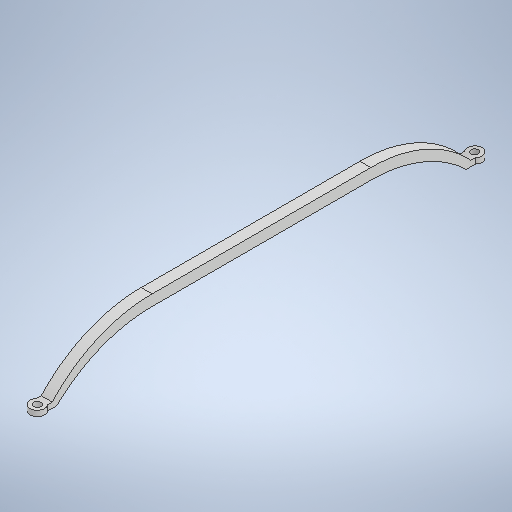
# Autodesk Inventor part: lacznik2
Saved by Autodesk Inventor 2025.2 (Build 292293000, 293)
## iProperties
Created: 2025-05-29
Part Number: lacznik2
Material: Ogólny
Document SubType Name: Modeling
Designer: janla
Density: 1 g/cm^3
Appearance: Domyślna
Author: janla
Autodesk Inventor part; units mm, degrees
ref_plane "YZ Plane" through (0, 0, 0) normal (1, 0, 0) x (0, 1, 0)
ref_plane "XZ Plane" through (0, 0, 0) normal (0, 1, 0) x (-1, 0, 0)
ref_plane "XY Plane" through (0, 0, 0) normal (0, 0, 1) x (1, 0, 0)
sketch "Szkic1" plane through (0, 0, 0) normal (0, 1, 0) x (-1, 0, 0)
  line L0 (0, 0) -> (0, -120)
  line L1 (0, -120) -> (0, 120)
  circle A0 centre (0, 120) radius 2
  circle A1 centre (0, -120) radius 2
  circle A2 centre (0, -120) radius 4
  circle A3 centre (0, 120) radius 4
  line L2 (-3, 117.3542) -> (3, 117.3542)
  line L3 (3, 117.3542) -> (3, -117.3542)
  line L4 (3, -117.3542) -> (-3, -117.3542)
  line L5 (-3, -117.3542) -> (-3, 117.3542)
  line L6 (3, 117.3542) -> (-3, 117.3542)
  line L7 (-3, 117.3542) -> (-3, 112.3542)
  line L8 (-3, 112.3542) -> (3, 112.3542)
  line L9 (3, 112.3542) -> (3, 117.3542)
  line L10 (3, -117.3542) -> (-3, -117.3542)
  line L11 (-3, -117.3542) -> (-3, -112.3542)
  line L12 (-3, -112.3542) -> (3, -112.3542)
  line L13 (3, -112.3542) -> (3, -117.3542)
  point P0 (-3, -117.3542)
  point P1 (3, -112.3542)
  point P2 (3, 112.3542)
  dimension "d4" = 8
  dimension "d5" = 8
  dimension "d0" = 120
  dimension "d1" = 240
  dimension "d2" = 4
  dimension "d3" = 4
  dimension "d6" = 3
  dimension "d7" = 3
  dimension "d14" = 5
  dimension "d15" = 5
  constraints: 28 end point, 6 parallel, 4 coincident, 3 horizontal, 3 perpendicular, 3 point on line, 2 centre point, 1 vertical, 6 other
  measures "d0" distance of L0.start L0.end
  measures "d1" distance of L0.end L1.end
  measures "d2" diameter of A0
  measures "d3" diameter of A1
  measures "d6" distance between parallel lines of L0 L5
  measures "d7" distance between parallel lines of L3 L0
  measures "d14" distance between parallel lines of L8 L2
  measures "d15" distance between parallel lines of L4 L12
extrude "Wyciągnięcie proste1" add sketch "Szkic1" along normal blind 3 contours L12 L3 A2 L0 | L0 A2 L5 L12 | L8 L5 A3 L1 | L1 A3 L3 L8 | A2 L4 L0 | L0 L4 A2 | A3 L2 L1 | L1 L2 A3 | L4 A2 | L2 A3
sketch "Szkic4" plane through (3, 0, 117.3542) normal (1, 0, 0) x (0, 0, -1)
  line L0 (0, 3) -> (5, 3) projected
  line L1 (2.5, 3) -> (232.2085, 3)
  line L2 (232.2085, 3) -> (117.3542, 3)
  line L3 (117.3542, 0) -> (117.3542, 27)
  line L4 (117.3542, 27) -> (177.3542, 27)
  line L5 (177.3542, 27) -> (57.3542, 27)
  arc A0 (57.3542, 27) -> (2.5, 3) centre (57.3542, -47.6873) ccw
  arc A1 (232.2085, 3) -> (177.3542, 27) centre (177.3542, -47.6873) ccw
  line L6 (57.3542, 27) -> (177.3542, 27)
  line L7 (177.3542, 27) -> (177.3542, 21)
  line L8 (177.3542, 21) -> (57.3542, 21)
  line L9 (57.3542, 21) -> (57.3542, 27)
  line L10 (0, 0) -> (5, 0) projected
  arc A2 (57.3542, 21) -> (5, 0) centre (57.3542, -54.7611) ccw
  line L11 (229.7085, 0) -> (229.7085, 3) projected
  arc A3 (229.7085, 0) -> (177.3542, 21) centre (177.3542, -54.7611) ccw
  line L12 (5, 0) -> (5, 3)
  point P0 (226.3787, 3)
  dimension "d26" = 27
  dimension "d27" = 60
  dimension "d28" = 120
  dimension "d29" = 6
  constraints: 20 end point, 8 point on circle, 4 centre point, 4 tangent, 2 horizontal, 2 midpoint, 2 parallel, 2 perpendicular, 2 vertical, 1 point on line
  measures "d26" distance of L3.start L3.end
  measures "d27" distance of L3.end L4.end
  measures "d28" distance of L4.end L5.end
  measures "d29" distance between parallel lines of L5 L8
extrude "Wyciągnięcie proste4" add sketch "Szkic4" against normal blind 6 contours A0 L9 A2 L1 L0 | L1 A2 L12 | L5 L3 L8 L9 | L4 L7 L8 L3 | A1 L1 A3 L7 | L1 L11 A3
